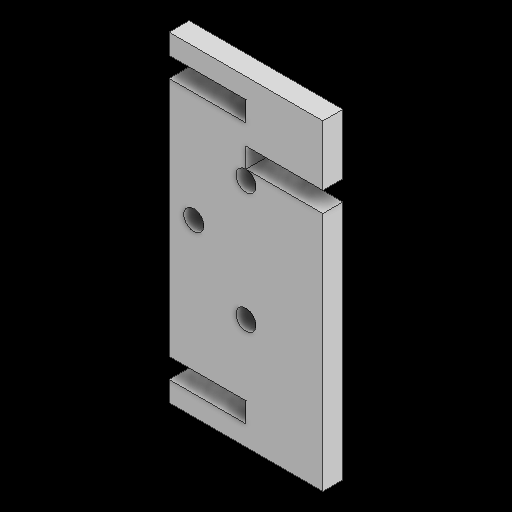
# Autodesk Inventor part: SoporteMotor
Saved by Autodesk Inventor 2025.2 (Build 292293000, 293)
## iProperties
Created: 2024-12-02
Part Number: SoporteMotor
Material: Generic
Document SubType Name: Modeling
Designer: braughton
Density: 1 g/cm^3
Appearance: Default
Author: braughton
Autodesk Inventor part; units mm, degrees
ref_plane "YZ Plane" through (0, 0, 0) normal (1, 0, 0) x (0, 1, 0)
ref_plane "XZ Plane" through (0, 0, 0) normal (0, 1, 0) x (-1, 0, 0)
ref_plane "XY Plane" through (0, 0, 0) normal (0, 0, 1) x (1, 0, 0)
sketch "Sketch2" plane through (0, 0, 0) normal (0, 0, 1) x (1, 0, 0)
  line L0 (63.1771, 54.6278) -> (40.1771, 54.6278)
  line L1 (40.1771, 51.6278) -> (51.6771, 51.6278)
  line L2 (51.6771, 51.6278) -> (51.6771, 48.6278)
  line L3 (51.6771, 48.6278) -> (40.1771, 48.6278)
  line L4 (51.6771, 45.6278) -> (63.1771, 45.6278)
  line L5 (63.1771, 45.6278) -> (63.1771, 45)
  line L6 (63.1771, 42.6278) -> (51.6771, 42.6278)
  line L7 (51.6771, 42.6278) -> (51.6771, 45.6278)
  line L8 (40.1771, 12.6278) -> (51.6771, 12.6278)
  line L9 (51.6771, 12.6278) -> (51.6771, 9.6278)
  line L10 (51.6771, 9.6278) -> (40.1771, 9.6278)
  line L11 (40.1771, 6.6278) -> (51.6771, 6.6278)
  line L12 (51.6771, 6.6278) -> (63.1771, 6.6278)
  circle A0 centre (51.6771, 41.1278) radius 1.5
  circle A1 centre (51.6771, 23.1278) radius 1.5
  circle A2 centre (43.8771, 32.1278) radius 1.5
  line L13 (40.1771, 9.6278) -> (40.1771, 6.6278)
  line L14 (40.1771, 54.6278) -> (40.1771, 51.6278)
  line L15 (40.1771, 48.6278) -> (40.1771, 12.6278)
  line L16 (63.1771, 6.6278) -> (63.1771, 42.6278)
  line L17 (63.1771, 45.6278) -> (63.1771, 54.6278)
  constraints: 36 end point, 2 centre point, 1 vertical alignment, 2 other
extrude "Extrusion1" add sketch "Sketch2" along normal blind 3
body "Solid1"
